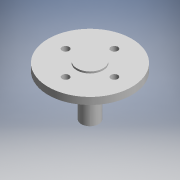
# Autodesk Inventor part: Servo_arm
Saved by Autodesk Inventor 2017 (Build 210142000, 142)
## iProperties
Part Number: Servo_arm
Material: ABS Plastic
Document SubType Name: Modeling
Designer: alex-
Appearance: White
Density: 1.06 g/cm^3
sa_diameter: 24,000 mm
sa_thickness: 2,000 mm
Author: alex-
Autodesk Inventor part; units mm, degrees
ref_plane "YZ Plane" through (0, 0, 0) normal (1, 0, 0) x (0, 1, 0)
ref_plane "XZ Plane" through (0, 0, 0) normal (0, 1, 0) x (-1, 0, 0)
ref_plane "XY Plane" through (0, 0, 0) normal (0, 0, 1) x (1, 0, 0)
sketch "Sketch1" plane through (0, 0, 0) normal (0, 1, 0) x (-1, 0, 0)
  circle A0 centre (0, 0) radius 12
  dimension "sa_diameter" = 24
  constraints: 1 centre point, 1 coincident
  measures "sa_diameter" diameter of A0
extrude "Extrusion1" add sketch "Sketch1" along normal blind 2
sketch "Sketch2" plane through (0, 0, 0) normal (0, -1, 0) x (1, 0, 0)
  circle A0 centre (0, 0) radius 2.5
  dimension "d4" = 5
  constraints: 1 centre point, 1 coincident
  measures "d4" diameter of A0
extrude "Extrusion2" add sketch "Sketch2" along normal blind 12
sketch "Sketch4" plane through (0, 2, 0) normal (0, 1, 0) x (1, 0, 0)
  circle A0 centre (0, 0) radius 3.75
  dimension "d12" = 7.5
  constraints: 1 centre point, 1 coincident
  measures "d12" diameter of A0
extrude "Extrusion4" add sketch "Sketch4" along normal blind 0.5
sketch "Sketch5" plane through (0, 2, 0) normal (0, 1, 0) x (1, 0, 0)
  circle A0 centre (0, 7) radius 1
  circle A1 centre (0, -7) radius 1
  circle A2 centre (-7, 0) radius 1
  circle A3 centre (7, 0) radius 1
  point P0 (0, 0)
  dimension "sa_hole_distance" = 7
  dimension "d16" = 7
  dimension "sa_hole_diameter" = 2
  dimension "d20" = 7
  dimension "d21" = 7
  constraints: 4 centre point, 3 equal radius, 2 horizontal alignment, 2 vertical alignment
  measures "sa_hole_distance" distance of point (0, 0) A0.centre
  measures "d16" distance of point (0, 0) A1.centre
  measures "sa_hole_diameter" diameter of A0
  measures "d20" distance of point (0, 0) A3.centre
  measures "d21" distance of point (0, 0) A2.centre
extrude "Extrusion5" cut sketch "Sketch5" against normal through all
equation "\"d16\" = sa_hole_distance"
equation "\"d20\" = sa_hole_distance"
equation "\"d21\" = sa_hole_distance"
body "Solid1"
